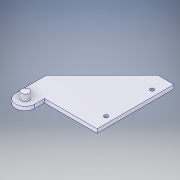
# Autodesk Inventor part: sideplateshaft_std
Saved by Autodesk Inventor 2017 (Build 210142000, 142)
## iProperties
Created: 2017-03-10
Part Number: sideplateshaft_std
Material: Generic
Document SubType Name: Modeling
Designer: Naga
Density: 1 g/cm^3
Appearance: Cool White
Author: Naga
Autodesk Inventor part; units mm, degrees
ref_plane "YZ Plane" through (0, 0, 0) normal (1, 0, 0) x (0, 1, 0)
ref_plane "XZ Plane" through (0, 0, 0) normal (0, 1, 0) x (-1, 0, 0)
ref_plane "XY Plane" through (0, 0, 0) normal (0, 0, 1) x (1, 0, 0)
sketch "Sketch3" plane through (0, 0, 0) normal (0, 1, 0) x (-1, 0, 0)
  line L0 (0, 0) -> (0, -60)
  line L1 (0, 0) -> (60, 0) construction
  line L2 (0, -60) -> (12.519, -60)
  line L3 (0, 0) -> (41, 0)
  line L4 (41, 0) -> (41, 7.5)
  line L5 (41, 7.5) -> (56, 7.5)
  circle A0 centre (48.5, 7.5) radius 7.5
  circle A1 centre (48.5, 7.5) radius 3
  line L6 (56, 7.5) -> (56, -16.519)
  line L7 (56, -16.519) -> (12.519, -60)
  line L8 (0, -30) -> (5, -30)
  line L9 (5, -60) -> (5, -48)
  line L10 (5, 0) -> (5, -12)
  circle A2 centre (5, -12) radius 1.5
  circle A3 centre (5, -48) radius 1.5
  dimension "d6" = 60
  dimension "d7" = 90
  dimension "d8" = 12.519
  dimension "d9" = 41
  dimension "d10" = 7.5
  dimension "d11" = 15
  dimension "d12" = 6
  dimension "d13" = 24.019
  dimension "d18" = 5
  dimension "d19" = 12
  dimension "d20" = 12
  dimension "d21" = 3
  dimension "d22" = 3
  constraints: 22 end point, 5 vertical, 4 horizontal, 3 centre point, 3 coincident, 3 point on line, 2 midpoint, 2 perpendicular, 1 horizontal alignment, 2 other
  measures "d6" distance of L0.start L0.end
  measures "d7" angle of L0 L1
  measures "d8" distance of L0.end L2.end
  measures "d9" distance of L0.start L3.end
  measures "d10" distance of L3.end L4.end
  measures "d11" distance of L4.end L5.end
  measures "d12" diameter of A1
  measures "d13" distance of L5.end L6.end
  measures "d18" distance of L8.start L8.end
  measures "d19" distance of L9.start L9.end
  measures "d20" distance of L10.start L10.end
  measures "d21" diameter of A2
  measures "d22" diameter of A3
extrude "Extrusion1" add sketch "Sketch3" along normal blind 3 contours L3 L4 A0 L6 L7 L2 L0 | A0 L5 A1 | L5 A1 A0 | L5 A1 picked at (49.4145, 6.796)
sketch "Sketch4" plane through (0, 0, 0) normal (0, -1, 0) x (1, 0, 0)
  line L0 (-51.5, 7.5) -> (-45.5, 7.5) projected
  line L1 (-45.5, 7.5) -> (-51.5, 7.5) projected
  circle A0 centre (-48.5, 7.5) radius 3
  point P0 (0, 0)
  constraints: 1 centre point, 1 midpoint
extrude "Extrusion2" add sketch "Sketch4" against normal blind 8
body "Solid1"
